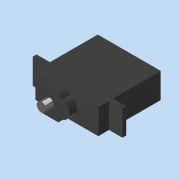
# Autodesk Inventor part: MiniServoBody
Saved by Autodesk Inventor 2017 (Build 210142000, 142)
## iProperties
Created: 2018-04-03
Part Number: MiniServoBody
Material: ABS Plastic
Document SubType Name: Modeling
Designer: Derek Wider
Density: 1.06 g/cm^3
Appearance: Smooth - Black
Author: Derek Wider
Autodesk Inventor part; units mm, degrees
ref_plane "YZ Plane" through (0, 0, 0) normal (1, 0, 0) x (0, 1, 0)
ref_plane "XZ Plane" through (0, 0, 0) normal (0, 1, 0) x (-1, 0, 0)
ref_plane "XY Plane" through (0, 0, 0) normal (0, 0, 1) x (1, 0, 0)
sketch "Sketch1" plane through (0, 0, 0) normal (0, 1, 0) x (-1, 0, 0)
  line L0 (0, 0) -> (29.718, 0)
  line L1 (29.718, 0) -> (29.718, -29.464)
  line L2 (29.718, -29.464) -> (0, -29.464)
  line L3 (0, -29.464) -> (0, 0)
  dimension "d0" = 29.718
  dimension "d1" = 29.464
  constraints: 8 end point, 2 parallel, 1 horizontal, 1 perpendicular
  measures "d0" distance of L1.end L2.end
  measures "d1" distance of L0.end L1.end
extrude "Extrusion1" add sketch "Sketch1" along normal blind 11.938
sketch "Sketch2" plane through (-29.718, 0, 0) normal (0, 0, 1) x (1, 0, 0)
  line L0 (29.718, 0) -> (0, 0) construction
  line L1 (29.718, 0) -> (29.718, 11.938) construction
  line L2 (0, 11.938) -> (29.718, 11.938) construction
  line L3 (0, 0) -> (0, 11.938) construction
  line L4 (0, 11.938) -> (29.718, 11.938) projected
  line L5 (5.715, 11.938) -> (15.875, 11.938)
  line L6 (15.875, 11.938) -> (15.875, 0)
  line L7 (15.875, 0) -> (5.715, 0)
  line L8 (5.715, 0) -> (5.715, 11.938)
  arc A0 (15.875, 2.0927) -> (15.875, 9.8453) centre (15.875, 5.969) ccw
  dimension "d4" = 10.16
  dimension "d5" = 5.715
  constraints: 8 end point, 4 point on line, 2 parallel, 2 point on circle, 1 centre point, 1 coincident, 1 horizontal, 1 line through centre, 1 midpoint, 1 perpendicular
  measures "d4" distance between parallel lines of L8 L6
  measures "d5" distance between parallel lines of L3 L8
extrude "Extrusion2" add sketch "Sketch2" along normal blind 3.81
sketch "Sketch3" plane through (-29.718, 0, 3.81) normal (0, 0, 1) x (1, 0, 0)
  line L0 (5.715, 11.938) -> (5.715, 0) construction
  line L1 (15.875, 11.938) -> (5.715, 11.938) construction
  circle A0 centre (10.414, 5.969) radius 2.159
  line L2 (15.875, 11.938) -> (15.875, 9.8453) projected
  arc A1 (15.875, 2.0927) -> (15.875, 9.8453) centre (15.875, 5.969) ccw projected
  line L3 (15.875, 2.0927) -> (15.875, 0) projected
  line L4 (29.718, 0) -> (15.875, 0) projected
  line L5 (29.718, 0) -> (29.718, 11.938) projected
  line L6 (15.875, 11.938) -> (29.718, 11.938) projected
  dimension "d8" = 4.318
  dimension "d18" = 19.304
  constraints: 1 centre point
  measures "d8" diameter of A0
  measures "d18" distance from line of A0.centre L5
extrude "Extrusion3" add sketch "Sketch3" along normal blind 3.81 contours A0
chamfer "Chamfer1" distance 1.27 angle 45 4 edges at (-24.003, 11.938, 1.905) (-13.843, 11.938, 1.905) (-24.003, 0, 1.905) (-13.843, 0, 1.905)
sketch "Sketch4" plane through (0, 11.938, 0) normal (0, 1, 0) x (1, 0, 0)
  line L0 (-15.113, 0) -> (0, 0) construction
  line L1 (0, 0) -> (0, 29.464) construction
  line L2 (0, 29.464) -> (-29.718, 29.464) construction
  line L3 (-29.718, 29.464) -> (-29.718, 0) construction
  line L4 (-29.718, 0) -> (-22.733, 0) construction
  line L5 (-22.733, -3.81) -> (-22.733, 0) construction
  line L6 (-15.113, -3.81) -> (-22.733, -3.81) construction
  line L7 (-15.113, 0) -> (-15.113, -3.81) construction
  line L8 (-29.718, 5.08) -> (-36.068, 5.08)
  line L9 (-36.068, 5.08) -> (-36.068, 6.8113)
  line L10 (-36.068, 6.8113) -> (-29.718, 6.8113)
  line L11 (-29.718, 6.8113) -> (-29.718, 5.08)
  line L12 (0, 5.08) -> (6.35, 5.08)
  line L13 (6.35, 5.08) -> (6.35, 6.8113)
  line L14 (6.35, 6.8113) -> (0, 6.8113)
  line L15 (0, 6.8113) -> (0, 5.08)
  dimension "d14" = 6.35
  dimension "d15" = 5.08
  constraints: 16 end point, 4 parallel, 4 point on line, 2 horizontal, 2 perpendicular, 1 collinear
  measures "d14" distance of L8.start L8.end
  measures "d15" distance between parallel lines of L8 L4
extrude "Extrusion4" add sketch "Sketch4" against normal up to surface (11.938 mm away)
body "Solid1"
